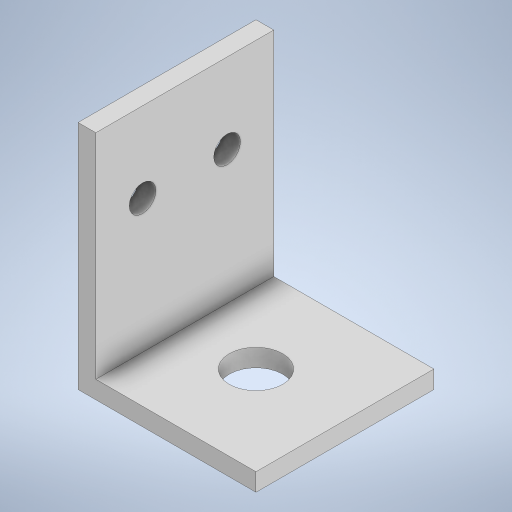
# Autodesk Inventor part: LimitSwitch MountV2
Saved by Autodesk Inventor 2023.2 (Build 272271030, 271C)
## iProperties
Created: 2023-05-02
Part Number: LimitSwitch MountV2
Material: Generic
Document SubType Name: Modeling
Designer: chase
Density: 1 g/cm^3
Appearance: Default
Author: chase
Autodesk Inventor part; units mm, degrees
ref_plane "YZ Plane" through (0, 0, 0) normal (1, 0, 0) x (0, 1, 0)
ref_plane "XZ Plane" through (0, 0, 0) normal (0, 1, 0) x (-1, 0, 0)
ref_plane "XY Plane" through (0, 0, 0) normal (0, 0, 1) x (1, 0, 0)
sketch "Sketch9" plane through (0, 0, 0) normal (0, 0, 1) x (1, 0, 0)
  line L0 (0, 0) -> (20, 0)
  line L1 (20, 0) -> (20, 26)
  line L2 (2, 26) -> (0, 26)
  line L3 (0, 26) -> (0, 0)
  line L4 (2, 26) -> (2, 2)
  line L5 (2, 2) -> (20, 2)
  line L6 (20, 2) -> (20, 26)
  dimension "d35" = 20
  dimension "d36" = 26
  dimension "d37" = 2
  dimension "d38" = 2
  constraints: 14 end point, 3 parallel, 1 horizontal, 1 perpendicular
  measures "d35" distance of L2.end L1.end
  measures "d36" distance of L1.end L0.end
  measures "d37" distance between parallel lines of L3 L4
  measures "d38" distance between parallel lines of L0 L5
extrude "Extrusion9" add sketch "Sketch9" against normal blind 20
sketch "Sketch10" plane through (0, 0, 0) normal (0, -1, 0) x (1, 0, 0)
  line L0 (0, 0) -> (20, 0) projected
  line L1 (10, 0) -> (10, -20)
  line L2 (20, -20) -> (0, -20) projected
  circle A0 centre (10, -10) radius 3
  dimension "d41" = 6
  constraints: 3 midpoint, 2 end point, 1 centre point
  measures "d41" diameter of A0
extrude "Extrusion10" cut sketch "Sketch10" against normal through all
sketch "Sketch11" plane through (0, 0, 0) normal (-1, 0, 0) x (0, 0, 1)
  line L0 (0, 26) -> (0, 0) projected
  line L1 (0, 26) -> (0, 17)
  circle A0 centre (-5.25, 17) radius 1.5
  circle A1 centre (-14.75, 17) radius 1.5
  dimension "d44" = 9
  dimension "d45" = 3
  dimension "d46" = 3
  dimension "d47" = 9.5
  dimension "d48" = 5.25
  constraints: 2 centre point, 2 end point, 1 point on line
  measures "d44" distance of L0.start L1.end
  measures "d45" diameter of A0
  measures "d46" diameter of A1
  measures "d47" distance of A1.centre A0.centre
  measures "d48" distance from line of L0 A0.centre
extrude "Extrusion11" cut sketch "Sketch11" against normal through all
body "Solid2"
